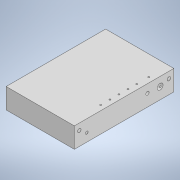
# Autodesk Inventor part: UBIQUITI EDGEROUTER-X
Saved by Autodesk Inventor 2020.2 (Build 242310000, 310)
## iProperties
Created: 2020-02-16
Part Number: UBIQUITI EDGEROUTER-X
Material: Generic
Document SubType Name: Modeling
Designer: mulve
Density: 1 g/cm^3
Appearance: Default
Author: mulve
Autodesk Inventor part; units mm, degrees
ref_plane "YZ Plane" through (0, 0, 0) normal (1, 0, 0) x (0, 1, 0)
ref_plane "XZ Plane" through (0, 0, 0) normal (0, 1, 0) x (-1, 0, 0)
ref_plane "XY Plane" through (0, 0, 0) normal (0, 0, 1) x (1, 0, 0)
sketch "Sketch1" plane through (0, 0, 0) normal (0, 1, 0) x (-1, 0, 0)
  line L0 (0, 0) -> (75.65, 0)
  line L1 (75.65, 0) -> (75.65, -110.31)
  line L2 (75.65, -110.31) -> (0, -110.31)
  line L3 (0, -110.31) -> (0, 0)
  dimension "d0" = 110.31
  dimension "d1" = 75.65
  constraints: 8 end point, 2 parallel, 1 horizontal, 1 perpendicular
  measures "d0" distance of L2.end L0.start
  measures "d1" distance of L1.end L2.end
extrude "Extrusion1" add sketch "Sketch1" along normal blind 22.5
sketch "Sketch2" plane through (0, 0, 0) normal (1, 0, 0) x (0, 0, -1)
  line L0 (0, 22.5) -> (110.31, 22.5) projected
  line L1 (0, 0) -> (0, 22.5) projected
  line L2 (110.31, 0) -> (110.31, 22.5) projected
  circle A0 centre (5.54, 15.27) radius 1.925
  circle A1 centre (104.77, 15.27) radius 1.925
  dimension "d4" = 7.23
  dimension "d5" = 7.23
  dimension "d6" = 5.54
  dimension "d7" = 5.54
  dimension "d8" = 3.85
  constraints: 2 centre point, 2 coincident, 1 equal radius
  measures "d4" distance from line of L0 point (5.54, 15.27)
  measures "d5" distance from line of L0 point (104.77, 15.27)
  measures "d6" distance from line of L1 point (5.54, 15.27)
  measures "d7" distance from line of L2 point (104.77, 15.27)
  measures "d8" diameter of A0
extrude "Extrusion2" cut sketch "Sketch2" against normal blind 0.1
sketch "Sketch3" plane through (0, 0, 0) normal (1, 0, 0) x (0, 0, -1)
  line L0 (0, 22.5) -> (110.31, 22.5) projected
  line L1 (0, 0) -> (0, 22.5) projected
  circle A0 centre (81.06, 13.3) radius 1.875
  dimension "d11" = 9.2
  dimension "d12" = 81.06
  dimension "d13" = 3.75
  constraints: 1 centre point, 1 coincident
  measures "d11" distance from line of L0 point (81.06, 13.3)
  measures "d12" distance from line of L1 point (81.06, 13.3)
  measures "d13" diameter of A0
extrude "Extrusion3" cut sketch "Sketch3" against normal blind 12.7
sketch "Sketch4" plane through (0, 0, 0) normal (1, 0, 0) x (0, 0, -1)
  line L0 (0, 0) -> (0, 22.5) projected
  line L1 (0, 22.5) -> (110.31, 22.5) projected
  circle A0 centre (13.8, 9.13) radius 1.5
  dimension "d16" = 13.8
  dimension "d17" = 13.37
  dimension "d18" = 3
  constraints: 1 centre point, 1 coincident
  measures "d16" distance from line of L0 point (13.8, 9.13)
  measures "d17" distance from line of L1 point (13.8, 9.13)
  measures "d18" diameter of A0
extrude "Extrusion4" cut sketch "Sketch4" against normal blind 0.2
sketch "Sketch5" plane through (0, 0, 0) normal (1, 0, 0) x (0, 0, -1)
  line L0 (90.8, 16.86) -> (99.47, 16.86)
  line L1 (99.47, 16.86) -> (99.47, 5.38)
  line L2 (99.47, 5.38) -> (90.8, 5.38)
  line L3 (90.8, 5.38) -> (90.8, 16.86)
  line L4 (110.31, 0) -> (110.31, 22.5) projected
  line L5 (0, 22.5) -> (110.31, 22.5) projected
  circle A0 centre (95.135, 12.62) radius 3.24
  circle A1 centre (95.135, 12.62) radius 1.125
  point P0 (0, 0)
  point P1 (95.135, 15.86)
  dimension "d25" = 6.48
  dimension "d21" = 8.67
  dimension "d22" = 10.84
  dimension "d23" = 11.48
  dimension "d24" = 5.64
  dimension "d26" = 1
  dimension "d27" = 2.25
  constraints: 8 end point, 2 coincident, 2 parallel, 1 centre point, 1 horizontal, 1 perpendicular, 1 vertical alignment, 2 other
  measures "d21" distance of L1.end L2.end
  measures "d22" distance between parallel lines of L4 L1
  measures "d23" distance of L0.end L1.end
  measures "d24" distance between parallel lines of L5 L0
  measures "d26" distance from line of L0 point (95.135, 15.86)
  measures "d27" diameter of A1
extrude "Extrusion5" cut sketch "Sketch5" against normal blind 9.2 contours A0
sketch "Sketch7" plane through (-75.65, 0, -110.31) normal (-1, 0, 0) x (0, 0, 1)
  line L0 (8.57, 5.39) -> (25.73, 5.39)
  line L1 (25.73, 5.39) -> (25.73, 19.5)
  line L2 (25.73, 19.5) -> (8.57, 19.5)
  line L3 (8.57, 19.5) -> (8.57, 5.39)
  line L4 (0, 22.5) -> (110.31, 22.5) projected
  line L5 (0, 0) -> (0, 22.5) projected
  line L6 (44.78, 5.39) -> (44.78, 19.5)
  line L7 (44.78, 19.5) -> (27.62, 19.5)
  line L8 (27.62, 19.5) -> (27.62, 5.39)
  line L9 (27.62, 5.39) -> (44.78, 5.39)
  line L10 (63.83, 5.39) -> (63.83, 19.5)
  line L11 (63.83, 19.5) -> (46.67, 19.5)
  line L12 (46.67, 19.5) -> (46.67, 5.39)
  line L13 (46.67, 5.39) -> (63.83, 5.39)
  line L14 (82.88, 5.39) -> (82.88, 19.5)
  line L15 (82.88, 19.5) -> (65.72, 19.5)
  line L16 (65.72, 19.5) -> (65.72, 5.39)
  line L17 (65.72, 5.39) -> (82.88, 5.39)
  line L18 (101.93, 5.39) -> (101.93, 19.5)
  line L19 (101.93, 19.5) -> (84.77, 19.5)
  line L20 (84.77, 19.5) -> (84.77, 5.39)
  line L21 (84.77, 5.39) -> (101.93, 5.39)
  point P0 (110.31, 0)
  dimension "d30" = 17.16
  dimension "d31" = 14.11
  dimension "d32" = 3
  dimension "d33" = 8.57
  dimension "d36" = 19.05
  constraints: 40 end point, 2 horizontal, 2 parallel, 1 perpendicular, 32 other
  measures "d30" distance of L1.end L2.end
  measures "d31" distance of L0.end L1.end
  measures "d32" distance between parallel lines of L4 L2
  measures "d33" distance between parallel lines of L5 L3
  measures "d36" distance of L0.end L6.start
extrude "Extrusion6" cut sketch "Sketch7" against normal blind 0.1
sketch "Sketch8" plane through (-75.55, 0, -110.31) normal (-1, 0, 0) x (0, 0, 1)
  line L0 (11.1, 7.46) -> (23.2, 7.46)
  line L1 (23.2, 7.46) -> (23.2, 14.99)
  line L2 (23.2, 14.99) -> (11.1, 14.99)
  line L3 (11.1, 14.99) -> (11.1, 7.46)
  line L4 (8.57, 5.39) -> (8.57, 19.5) projected
  line L5 (25.73, 19.5) -> (25.73, 5.39) projected
  line L6 (25.73, 5.39) -> (8.57, 5.39) projected
  line L7 (13.815, 7.46) -> (20.485, 7.46)
  line L8 (20.485, 7.46) -> (20.485, 16.67)
  line L9 (20.485, 16.67) -> (13.815, 16.67)
  line L10 (13.815, 16.67) -> (13.815, 7.46)
  line L11 (15.055, 7.46) -> (19.245, 7.46)
  line L12 (19.245, 7.46) -> (19.245, 18.23)
  line L13 (19.245, 18.23) -> (15.055, 18.23)
  line L14 (15.055, 18.23) -> (15.055, 7.46)
  line L15 (34.155, 18.23) -> (34.155, 7.46)
  line L16 (30.2, 14.99) -> (30.2, 7.46)
  line L17 (32.915, 16.67) -> (32.915, 7.46)
  line L18 (38.345, 7.46) -> (38.345, 18.23)
  line L19 (39.585, 7.46) -> (39.585, 16.67)
  line L20 (42.3, 7.46) -> (42.3, 14.99)
  line L21 (38.345, 18.23) -> (34.155, 18.23)
  line L22 (39.585, 16.67) -> (32.915, 16.67)
  line L23 (42.3, 14.99) -> (30.2, 14.99)
  line L24 (34.155, 7.46) -> (38.345, 7.46)
  line L25 (30.2, 7.46) -> (42.3, 7.46)
  line L26 (53.255, 18.23) -> (53.255, 7.46)
  line L27 (49.3, 14.99) -> (49.3, 7.46)
  line L28 (52.015, 16.67) -> (52.015, 7.46)
  line L29 (57.445, 7.46) -> (57.445, 18.23)
  line L30 (58.685, 7.46) -> (58.685, 16.67)
  line L31 (61.4, 7.46) -> (61.4, 14.99)
  line L32 (57.445, 18.23) -> (53.255, 18.23)
  line L33 (58.685, 16.67) -> (52.015, 16.67)
  line L34 (61.4, 14.99) -> (49.3, 14.99)
  line L35 (53.255, 7.46) -> (57.445, 7.46)
  line L36 (49.3, 7.46) -> (61.4, 7.46)
  line L37 (72.355, 18.23) -> (72.355, 7.46)
  line L38 (68.4, 14.99) -> (68.4, 7.46)
  line L39 (71.115, 16.67) -> (71.115, 7.46)
  line L40 (76.545, 7.46) -> (76.545, 18.23)
  line L41 (77.785, 7.46) -> (77.785, 16.67)
  line L42 (80.5, 7.46) -> (80.5, 14.99)
  line L43 (76.545, 18.23) -> (72.355, 18.23)
  line L44 (77.785, 16.67) -> (71.115, 16.67)
  line L45 (80.5, 14.99) -> (68.4, 14.99)
  line L46 (72.355, 7.46) -> (76.545, 7.46)
  line L47 (68.4, 7.46) -> (80.5, 7.46)
  line L48 (91.455, 18.23) -> (91.455, 7.46)
  line L49 (87.5, 14.99) -> (87.5, 7.46)
  line L50 (90.215, 16.67) -> (90.215, 7.46)
  line L51 (95.645, 7.46) -> (95.645, 18.23)
  line L52 (96.885, 7.46) -> (96.885, 16.67)
  line L53 (99.6, 7.46) -> (99.6, 14.99)
  line L54 (95.645, 18.23) -> (91.455, 18.23)
  line L55 (96.885, 16.67) -> (90.215, 16.67)
  line L56 (99.6, 14.99) -> (87.5, 14.99)
  line L57 (91.455, 7.46) -> (95.645, 7.46)
  line L58 (87.5, 7.46) -> (99.6, 7.46)
  point P0 (110.31, 0)
  point P1 (91.455, 16.67)
  point P2 (90.215, 14.99)
  point P3 (91.455, 7.46)
  point P4 (96.885, 14.99)
  point P5 (95.645, 16.67)
  point P6 (77.785, 14.99)
  point P7 (76.545, 16.67)
  point P8 (72.355, 16.67)
  point P9 (71.115, 14.99)
  point P10 (72.355, 7.46)
  point P11 (53.255, 7.46)
  point P12 (58.685, 14.99)
  point P13 (57.445, 16.67)
  point P14 (53.255, 16.67)
  point P15 (52.015, 14.99)
  point P16 (39.585, 14.99)
  point P17 (38.345, 16.67)
  point P18 (34.155, 16.67)
  point P19 (32.915, 14.99)
  point P20 (34.155, 7.46)
  point P21 (15.055, 16.67)
  point P22 (13.815, 14.99)
  point P23 (20.485, 14.99)
  point P24 (19.245, 16.67)
  dimension "d43" = 12.1
  dimension "d45" = 2.53
  dimension "d46" = 2.53
  dimension "d47" = 2.07
  dimension "d48" = 6.67
  dimension "d50" = 2.715
  dimension "d51" = 2.715
  dimension "d52" = 4.19
  dimension "d53" = 12.84
  dimension "d54" = 11.28
  dimension "d55" = 9.6
  dimension "d56" = 1.24
  dimension "d57" = 1.24
  dimension "d60" = 19.1
  constraints: 112 end point, 6 parallel, 6 point on line, 4 horizontal, 3 perpendicular, 1 collinear, 91 other
  measures "d43" distance of L0.start L0.end
  measures "d45" distance between parallel lines of L4 L3
  measures "d46" distance between parallel lines of L5 L1
  measures "d47" distance between parallel lines of L6 L0
  measures "d48" distance of L8.end L9.end
  measures "d50" distance between parallel lines of L3 L10
  measures "d51" distance between parallel lines of L1 L8
  measures "d52" distance of L12.end L13.end
  measures "d53" distance between parallel lines of L6 L13
  measures "d54" distance between parallel lines of L6 L9
  measures "d55" distance between parallel lines of L6 L2
  measures "d56" distance between parallel lines of L10 L14
  measures "d57" distance between parallel lines of L8 L12
  measures "d60" distance of L13.end L15.start
extrude "Extrusion7" cut sketch "Sketch8" against normal blind 15.75
sketch "Sketch9" plane through (0, 22.5, 0) normal (0, 1, 0) x (1, 0, 0)
  line L0 (0, 0) -> (0, 110.31) projected
  line L1 (0, 110.31) -> (-75.65, 110.31) projected
  circle A0 centre (-5.6, 88.05) radius 0.83
  circle A1 centre (-5.6, 74.79) radius 0.83
  circle A2 centre (-5.6, 65.06) radius 0.83
  circle A3 centre (-5.6, 55) radius 0.83
  circle A4 centre (-5.6, 45.05) radius 0.83
  circle A5 centre (-5.6, 34.75) radius 0.83
  dimension "d67" = 5.6
  dimension "d68" = 5.6
  dimension "d69" = 5.6
  dimension "d70" = 5.6
  dimension "d71" = 5.6
  dimension "d72" = 22.26
  dimension "d73" = 35.52
  dimension "d74" = 45.25
  dimension "d75" = 55.31
  dimension "d76" = 65.26
  dimension "d77" = 5.6
  dimension "d78" = 75.56
  dimension "d79" = 1.66
  constraints: 6 centre point, 6 coincident, 5 equal radius
  measures "d67" distance from line of L0 point (-5.6, 88.05)
  measures "d68" distance from line of L0 point (-5.6, 74.79)
  measures "d69" distance from line of L0 point (-5.6, 65.06)
  measures "d70" distance from line of L0 point (-5.6, 55)
  measures "d71" distance from line of L0 point (-5.6, 45.05)
  measures "d72" distance from line of L1 point (-5.6, 88.05)
  measures "d73" distance from line of L1 point (-5.6, 74.79)
  measures "d74" distance from line of L1 point (-5.6, 65.06)
  measures "d75" distance from line of L1 point (-5.6, 55)
  measures "d76" distance from line of L1 point (-5.6, 45.05)
  measures "d77" distance from line of L0 point (-5.6, 34.75)
  measures "d78" distance from line of L1 point (-5.6, 34.75)
  measures "d79" diameter of A0
extrude "Extrusion8" cut sketch "Sketch9" against normal blind 0.1
sketch "Sketch10" plane through (0, 0, 0) normal (0, -1, 0) x (1, 0, 0)
  line L0 (0, 0) -> (0, -110.31) projected
  line L1 (-75.65, 0) -> (0, 0) projected
  circle A0 centre (-9.5, -13.8) radius 4.3
  circle A1 centre (-9.5, -95.08) radius 4.3
  circle A2 centre (-55.22, -13.8) radius 4.3
  circle A3 centre (-55.22, -95.08) radius 4.3
  dimension "d82" = 9.5
  dimension "d83" = 13.8
  dimension "d84" = 8.6
  dimension "d87" = 81.28
  dimension "d90" = 45.72
  constraints: 4 centre point, 1 coincident, 1 horizontal, 1 vertical, 6 other
  measures "d82" distance from line of L0 point (-9.5, -13.8)
  measures "d83" distance from line of L1 point (-9.5, -13.8)
  measures "d84" diameter of A0
  measures "d87" distance of A0.centre A1.centre
  measures "d90" distance of A0.centre A2.centre
extrude "Extrusion9" cut sketch "Sketch10" against normal blind 0.33
sketch "Sketch11" plane through (-9.5, 0.33, -13.8) normal (0, -1, 0) x (1, 0, 0)
  circle A0 centre (0, 0) radius 3.825
  line L0 (9.5, 13.8) -> (9.5, -96.51) projected
  line L1 (9.5, -26.4546) -> (9.5, -62.5532)
  line L2 (-14.9441, 13.8) -> (-34.0604, 13.8)
  circle A1 centre (0, -81.3) radius 3.825
  circle A2 centre (-45.7, 0) radius 3.825
  circle A3 centre (-45.7, -81.3) radius 3.825
  dimension "d95" = 7.65
  dimension "d98" = 81.3
  dimension "d101" = 45.7
  constraints: 4 centre point, 4 end point, 2 horizontal, 2 point on line, 1 vertical, 6 other
  measures "d95" diameter of A0
  measures "d98" distance of A0.centre A1.centre
  measures "d101" distance of A0.centre A2.centre
extrude "Extrusion10" add sketch "Sketch11" along normal blind 1.91
fillet "Fillet1" radius 3.82 4 edges at (-13.325, -1.58, -13.8) (-59.025, -1.58, -13.8) (-13.325, -1.58, -95.1) (-59.025, -1.58, -95.1)
equation "\"d45\" = d46"
equation "\"d50\" = d51"
equation "\"d56\" = d57"
equation "\"d68\" = d67"
equation "\"d69\" = d68"
equation "\"d70\" = d69"
equation "\"d71\" = d70"
equation "\"d77\" = d71"
body "Solid1"
